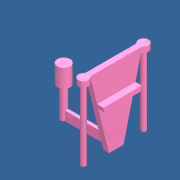
# Autodesk Inventor part: Cube Cage
Saved by Autodesk Inventor 2020 (Build 240168000, 168)
## iProperties
Created: 2019-12-14
Part Number: Cube Cage
Material: ABS Plastic
Document SubType Name: Modeling
Designer: Jack
Density: 1.06 g/cm^3
Appearance: Smooth - White
Author: Jack
Autodesk Inventor part; units mm, degrees
ref_plane "YZ Plane" through (0, 0, 0) normal (1, 0, 0) x (0, 1, 0)
ref_plane "XZ Plane" through (0, 0, 0) normal (0, 1, 0) x (-1, 0, 0)
ref_plane "XY Plane" through (0, 0, 0) normal (0, 0, 1) x (1, 0, 0)
sketch "Sketch1" plane through (0, 0, 0) normal (0, 1, 0) x (-1, 0, 0)
  circle A0 centre (0, 0) radius 3.5
  dimension "d0" = 7
  constraints: 1 centre point, 1 coincident
  measures "d0" diameter of A0
extrude "Extrusion1" add sketch "Sketch1" along normal blind 33
sketch "Sketch2" plane through (0, 33, 0) normal (0, 1, 0) x (1, 0, 0)
  circle A0 centre (0, 0) radius 7
  dimension "d3" = 14
  constraints: 1 centre point, 1 coincident
  measures "d3" diameter of A0
extrude "Extrusion2" add sketch "Sketch2" along normal blind 20
sketch "Sketch3" plane through (0, 0, 0) normal (0, 0, 1) x (1, 0, 0)
  line L0 (0, 0) -> (57.5, 0)
  line L1 (57.5, 0) -> (57.5, 10)
  line L2 (57.5, 10) -> (0, 10)
  line L3 (0, 10) -> (0, 0)
  dimension "d6" = 57.5
  dimension "d7" = 10
  constraints: 8 end point, 2 parallel, 1 horizontal, 1 perpendicular
  measures "d6" distance of L1.end L2.end
  measures "d7" distance of L0.end L1.end
extrude "Extrusion3" add sketch "Sketch3" along normal mid plane 3.5
sketch "Sketch4" plane through (57.5, 0, 1.75) normal (1, 0, 0) x (0, 0, -1)
  line L0 (1.75, 0) -> (9.75, 0)
  line L1 (9.75, 0) -> (28.75, 77)
  line L2 (1.75, 0) -> (1.75, 77)
  line L3 (1.75, 77) -> (28.75, 77)
  dimension "d10" = 8
  dimension "d11" = 27
  dimension "d12" = 77
  constraints: 8 end point, 1 horizontal, 1 parallel, 1 vertical
  measures "d10" distance of L0.start L0.end
  measures "d11" distance of L2.end L1.end
  measures "d12" distance of L0.start L2.end
extrude "Extrusion4" add sketch "Sketch4" against normal blind 6
sketch "Sketch5" plane through (57.5, 77, 0) normal (0, 1, 0) x (1, 0, 0)
  line L0 (0, 27) -> (0, 0) projected
  line L1 (0, 27) -> (-6, 27) projected
  line L2 (-6, 0) -> (-6, 27) projected
  line L3 (0, 0) -> (-6, 0) projected
  point P0 (-57.5, 0)
extrude "Extrusion5" add sketch "Sketch5" along normal blind 6
sketch "Sketch6" plane through (57.5, 83, 0) normal (0, 1, 0) x (1, 0, 0)
  circle A0 centre (-3, 33) radius 5.5
  line L0 (-6, 0) -> (0, 0) projected
  line L1 (-6, 27) -> (-6, 0) projected
  line L2 (-6, 27) -> (-8.5, 33)
  line L3 (0, 8) -> (0, 27) projected
  line L4 (0, 27) -> (2.5, 33)
  line L5 (0, 27) -> (-6, 27) projected
  line L6 (-6, 27) -> (0, 27)
  line L7 (-8.5, 33) -> (2.5, 33)
  point P0 (-57.5, 0)
  point P1 (0.8728, 29.0947)
  point P2 (-6.8728, 29.0947)
  dimension "d17" = 11
  dimension "d18" = 33
  dimension "d19" = 3
  constraints: 8 end point, 2 point on circle, 1 centre point, 1 collinear, 1 horizontal
  measures "d17" diameter of A0
  measures "d18" distance from line of L0 A0.centre
  measures "d19" distance from line of L1 A0.centre
extrude "Extrusion6" add sketch "Sketch6" against normal blind 6
sketch "Sketch7" plane through (57.5, 77, 0) normal (0, -1, 0) x (1, 0, 0)
  arc A0 (-6.8728, -29.0947) -> (0.8728, -29.0947) centre (-3, -33) ccw projected
  circle A1 centre (-3, -33) radius 2.75
  point P0 (-57.5, 0)
  dimension "d22" = 5.5
  constraints: 1 centre point, 1 coincident
  measures "d22" diameter of A1
extrude "Extrusion7" add sketch "Sketch7" along normal blind 77
mirror "Mirror1" about plane through (57.5, 0, 0) normal (0, 0, 1) of "Extrusion4", "Extrusion6", "Extrusion5", "Extrusion7"
sketch "Sketch8" plane through (57.5, 77, -27) normal (1, 0, 0) x (0, 0, -1)
  line L0 (-27, -77) -> (-27, -3.2697)
  line L1 (-46.8442, -29) -> (-7.1558, -29)
  line L2 (-7.1558, -29) -> (-5.9221, -24)
  line L3 (-5.9221, -24) -> (-48.0779, -24)
  line L4 (-48.0779, -24) -> (-46.8442, -29)
  line L5 (-46.8442, -29) -> (-5.9221, -24) construction
  line L6 (-7.1558, -29) -> (-48.0779, -24) construction
  line L7 (0, 6) -> (-54, 6) projected
  line L8 (-19, -77) -> (0, 0) projected
  line L9 (-35, -77) -> (-54, 0) projected
  point P0 (-27, -26.5754)
  dimension "d27" = 30
  dimension "d30" = 5
  constraints: 14 end point, 3 point on line, 2 collinear, 1 horizontal, 1 parallel, 1 vertical
  measures "d27" distance between parallel lines of L7 L3
  measures "d30" vertical distance of L1.end L2.end
extrude "Extrusion8" add sketch "Sketch8" along normal blind 7
sketch "Sketch10" plane through (0, 53, 0) normal (0, 1, 0) x (1, 0, 0)
  line L0 (25, 2.5) -> (-25, 2.5)
  line L1 (-25, 2.5) -> (-25, -2.5)
  line L2 (-25, -2.5) -> (25, -2.5)
  line L3 (25, -2.5) -> (25, 2.5)
  line L4 (25, 2.5) -> (-25, -2.5) construction
  line L5 (-25, 2.5) -> (25, -2.5) construction
  point P0 (0, 0)
  dimension "d31" = 50
  dimension "d32" = 5
  constraints: 12 end point, 2 midpoint, 2 parallel, 1 horizontal, 1 perpendicular
  measures "d31" distance of L1.end L2.end
  measures "d32" distance of L0.end L1.end
extrude "Extrusion9" add sketch "Sketch10" against normal blind 20
chamfer "Chamfer1" distance 15 angle 45 2 edges at (25, 33, 0) (-25, 33, 0)
fillet "Fillet1" radius 2 4 edges at (15.7692, 53, -2.5) (-15.7692, 53, -2.5) (-15.7692, 53, 2.5) (15.7692, 53, 2.5)
body "Solid1"
